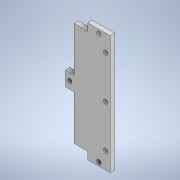
# Autodesk Inventor part: side steel plates
Saved by Autodesk Inventor 2022 (Build 260153000, 153)
## iProperties
Created: 2023-03-21
Part Number: side steel plates
Material: Generic
Document SubType Name: Modeling
Designer: chris
Density: 1 g/cm^3
Appearance: Default
Author: chris
Autodesk Inventor part; units mm, degrees
ref_plane "YZ Plane" through (0, 0, 0) normal (1, 0, 0) x (0, 1, 0)
ref_plane "XZ Plane" through (0, 0, 0) normal (0, 1, 0) x (-1, 0, 0)
ref_plane "XY Plane" through (0, 0, 0) normal (0, 0, 1) x (1, 0, 0)
sketch "Sketch1" plane through (0, 0, 0) normal (0, 0, 1) x (1, 0, 0)
  line L0 (0, 0) -> (18.5, 0)
  line L1 (0, 0) -> (0, 71)
  line L2 (0, 71) -> (18.5, 71)
  line L3 (18.5, 71) -> (18.5, 0)
  dimension "d0" = 18.5
  dimension "d1" = 71
  constraints: 8 end point, 2 horizontal, 1 perpendicular
  measures "d0" distance of L0.start L0.end
  measures "d1" distance of L0.start L1.end
extrude "Extrusion1" add sketch "Sketch1" along normal blind 3
sketch "Sketch2" plane through (0, 0, 3) normal (0, 0, 1) x (1, 0, 0)
  line L0 (0, 0) -> (18.5, 0) projected
  line L1 (18.5, 0) -> (18.5, 71) projected
  line L2 (18.5, 71) -> (0, 71) projected
  line L3 (0, 71) -> (0, 0) projected
  line L4 (24.5, 71) -> (24.5, 0)
  circle A0 centre (21.5, 64.5) radius 1.5
  circle A1 centre (21.5, 35.5) radius 1.5
  circle A2 centre (21.5, 6.5) radius 1.5
  line L5 (18.5, 71) -> (0, 71) projected
  line L6 (9.25, 71) -> (9.25, 76)
  line L7 (9.25, 76) -> (24.5, 76)
  line L8 (24.5, 76) -> (24.5, 71)
  circle A3 centre (16.875, 73.5) radius 1.5
  line L9 (0, 71) -> (0, 0) projected
  line L10 (9.25, 0) -> (9.25, -5)
  line L11 (9.25, -5) -> (24.5, -5)
  circle A4 centre (16.875, -2.5) radius 1.5
  line L12 (24.5, 0) -> (24.5, -5)
  dimension "d4" = 6
  dimension "d11" = 3
  dimension "d12" = 3
  dimension "d13" = 3
  dimension "d15" = 5
  constraints: 14 end point, 5 centre point, 2 perpendicular, 1 collinear, 1 midpoint, 1 vertical
  measures "d4" distance of L1.end L4.start
  measures "d11" diameter of A0
  measures "d12" diameter of A1
  measures "d13" diameter of A2
  measures "d15" distance of L6.start L6.end
extrude "Extrusion2" add sketch "Sketch2" against normal blind 3 contours L0 L1 L2 L6 L7 L8 L4 L12 L11 L10
sketch "Sketch3" plane through (0, 0, 3) normal (0, 0, 1) x (1, 0, 0)
  line L0 (0, 71) -> (0, 0) projected
  line L1 (0, 35.5) -> (-6, 35.5)
  line L2 (-6, 35.5) -> (-6, 30.5)
  line L3 (-6, 30.5) -> (0, 30.5)
  line L4 (-6, 35.5) -> (-6, 40.5)
  line L5 (-6, 40.5) -> (0, 40.5)
  circle A0 centre (-3, 35.5) radius 1.5
  dimension "d19" = 6
  dimension "d20" = 5
  dimension "d21" = 5
  dimension "d22" = 3
  constraints: 10 end point, 3 point on line, 2 midpoint, 2 perpendicular, 1 centre point, 1 horizontal, 1 vertical
  measures "d19" distance of L1.start L1.end
  measures "d20" distance of L1.end L2.end
  measures "d21" distance of L1.end L4.end
  measures "d22" diameter of A0
extrude "Extrusion3" add sketch "Sketch3" against normal blind 3 contours L0 L1 A0 L4 L5 | L0 L3 L2 L1 A0
body "Solid1"
